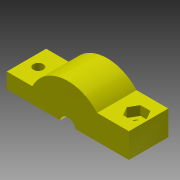
# Autodesk Inventor part: THREAD CLAMP
Saved by Autodesk Inventor 2013 (Build 170138000, 138)
## iProperties
Created: 2013-11-16
Part Number: THREAD CLAMP
Material: Generic
Document SubType Name: Modeling
Designer: employee
Density: 1 g/cm^3
Author: employee
Autodesk Inventor part; units mm, degrees
ref_plane "YZ Plane" through (0, 0, 0) normal (1, 0, 0) x (0, 1, 0)
ref_plane "XZ Plane" through (0, 0, 0) normal (0, 1, 0) x (-1, 0, 0)
ref_plane "XY Plane" through (0, 0, 0) normal (0, 0, 1) x (1, 0, 0)
sketch "Sketch1" plane through (0, 0, 0) normal (0, 0, 1) x (1, 0, 0)
  circle A0 centre (0, 0) radius 9.525 construction
  circle A1 centre (0, 0) radius 2.54 construction
  line L0 (-15.875, 0.5) -> (-2.4903, 0.5)
  line L1 (2.4903, 0.5) -> (15.875, 0.5)
  line L2 (15.875, 0.5) -> (15.875, 5.5)
  line L3 (15.875, 5.5) -> (7.7766, 5.5)
  line L4 (-15.875, 0.5) -> (-15.875, 5.5)
  line L5 (-15.875, 5.5) -> (-7.7766, 5.5)
  arc A2 (2.4903, 0.5) -> (-2.4903, 0.5) centre (0, 0) ccw
  arc A3 (7.7766, 5.5) -> (-7.7766, 5.5) centre (0, 0) ccw
  dimension "d0" = 5.08
  dimension "d2" = 19.05
  dimension "d3" = 0.5
  dimension "d4" = 5
  dimension "d5" = 15.875
  constraints: 12 end point, 8 point on circle, 4 centre point, 3 coincident, 3 perpendicular, 2 collinear, 2 horizontal alignment, 1 concentric, 1 horizontal, 1 parallel
  measures "d0" diameter of A1
  measures "d2" diameter of A0
  measures "d3" distance from line of L0 point (0, 0)
  measures "d4" distance of L0.start L4.end
  measures "d5" distance from line of L4 A2.centre
extrude "Extrusion1" add sketch "Sketch1" along normal blind 12.7
sketch "Sketch3" plane through (7.7766, 5.5, 0) normal (0, 1, 0) x (1, 0, 0)
  line L0 (8.0984, 0) -> (8.0984, -12.7) projected
  line L1 (-15.5532, 0) -> (0, 0) projected
  line L2 (-15.5532, 0) -> (-23.6516, 0) projected
  line L3 (-23.6516, 0) -> (-23.6516, -12.7) projected
  line L4 (-15.5532, -12.7) -> (-23.6516, -12.7) projected
  line L5 (-15.5532, 0) -> (-15.5532, -12.7) projected
  circle A0 centre (-19.6829, -6.35) radius 1.6
  circle A1 centre (4.1296, -6.35) radius 1.6
  point P0 (-7.7766, 0)
  point P1 (-23.6516, -6.35)
  point P2 (8.0984, -6.35)
  point P3 (-7.7766, 0)
  dimension "d13" = 3.2
  dimension "d15" = 11.9062
  dimension "d16" = 11.9062
  constraints: 2 centre point, 2 horizontal alignment, 2 midpoint, 1 coincident, 1 equal radius
  measures "d13" diameter of A0
  measures "d15" horizontal distance of A0.centre point (-7.777, 0)
  measures "d16" horizontal distance of A1.centre point (-7.777, 0)
extrude "Extrusion3" cut sketch "Sketch3" against normal through all contours A0 | A1
sketch "Sketch2" plane through (0, 0, 0) normal (0, 0, -1) x (-1, 0, 0)
  line L0 (15.875, 0.5) -> (2.4903, 0.5) projected
  line L1 (-2.4903, 0.5) -> (-15.875, 0.5) projected
  arc A0 (2.4903, 0.5) -> (-2.4903, 0.5) centre (0, 0) ccw projected
  arc A1 (7.9217, 0.5) -> (-7.9217, 0.5) centre (0, 0) ccw
  dimension "d8" = 7.9375
  constraints: 2 point on circle, 2 point on line, 1 centre point, 1 coincident
  measures "d8" radius of A1
extrude "Extrusion2" add sketch "Sketch2" along normal blind 1.5875
sketch "Sketch6" plane through (7.7766, 5.5, 0) normal (0, 1, 0) x (1, 0, 0)
  circle A0 centre (4.1296, -6.35) radius 1.6 projected
  line L0 (8.0984, 0) -> (0, 0) projected
  line L1 (8.0984, -12.7) -> (0, -12.7) projected
  line L2 (8.0984, 0) -> (8.0984, -12.7) projected
  line L3 (2.5131, -3.55) -> (5.7462, -3.55)
  line L4 (5.7462, -3.55) -> (7.3628, -6.35)
  line L5 (7.3628, -6.35) -> (5.7462, -9.15)
  line L6 (5.7462, -9.15) -> (2.5131, -9.15)
  line L7 (2.5131, -9.15) -> (0.8965, -6.35)
  line L8 (0.8965, -6.35) -> (2.5131, -3.55)
  line L9 (0, 0) -> (-8.0984, 0)
  line L10 (-8.0984, 0) -> (-8.0984, -12.7)
  line L11 (-8.0984, -12.7) -> (0, -12.7)
  line L12 (0, -12.7) -> (0, 0)
  point P0 (-7.7766, 0)
  dimension "d30" = 5.6
  constraints: 20 end point, 2 horizontal, 2 parallel, 1 coincident, 1 collinear, 1 perpendicular, 13 other
  measures "d30" distance between parallel lines of L4 L7
extrude "Extrusion5" add sketch "Sketch6" along normal blind 3 contours L2 L1 L12 L0 | L12 L11 L10 L9
equation "\"d16\" = d15"
body "Solid1"
